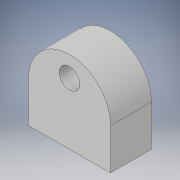
# Autodesk Inventor part: Scissor Anchor
Saved by Autodesk Inventor 2018 (Build 220112000, 112)
## iProperties
Created: 2018-01-18
Part Number: Scissor Anchor
Material: Generic
Document SubType Name: Modeling
Designer: Apple
Density: 1 g/cm^3
Appearance: Default
Author: Apple
Autodesk Inventor part; units mm, degrees
ref_plane "YZ Plane" through (0, 0, 0) normal (1, 0, 0) x (0, 1, 0)
ref_plane "XZ Plane" through (0, 0, 0) normal (0, 1, 0) x (-1, 0, 0)
ref_plane "XY Plane" through (0, 0, 0) normal (0, 0, 1) x (1, 0, 0)
sketch "Sketch1" plane through (0, 0, 0) normal (0, 0, 1) x (1, 0, 0)
  line L0 (-25.4, -12.7) -> (25.4, -12.7)
  line L1 (25.4, -12.7) -> (25.4, 12.7)
  line L2 (0, 38.1) -> (0, 38.1)
  line L3 (-25.4, 12.7) -> (-25.4, -12.7)
  circle A0 centre (0, 25.4) radius 6.35
  arc A1 (0, 38.1) -> (-25.4, 12.7) centre (0, 12.7) ccw
  arc A2 (25.4, 12.7) -> (0, 38.1) centre (0, 12.7) ccw
  point P0 (0, 0)
  point P1 (25.4, 38.1)
  point P2 (-25.4, 38.1)
  point P3 (-25.4, 0)
  point P4 (0, 38.1)
  dimension "d0" = 50.8
  dimension "d1" = 50.8
  dimension "d5" = 12.7
  dimension "d6" = 25.4
  dimension "d8" = 25.4
  constraints: 8 end point, 4 point on circle, 4 point on line, 4 tangent, 3 centre point, 2 midpoint, 2 parallel, 2 vertical alignment, 1 concentric, 1 horizontal, 1 horizontal alignment, 1 perpendicular
  measures "d0" distance of point (-25.4, 38.1) point (25.4, 38.1)
  measures "d1" distance of point (25.4, 38.1) L0.end
  measures "d5" diameter of A0
  measures "d6" distance of point (0, 0) A0.centre
  measures "d8" radius of A1
extrude "Extrusion2" add sketch "Sketch1" along normal blind 25.4
body "Solid2"
